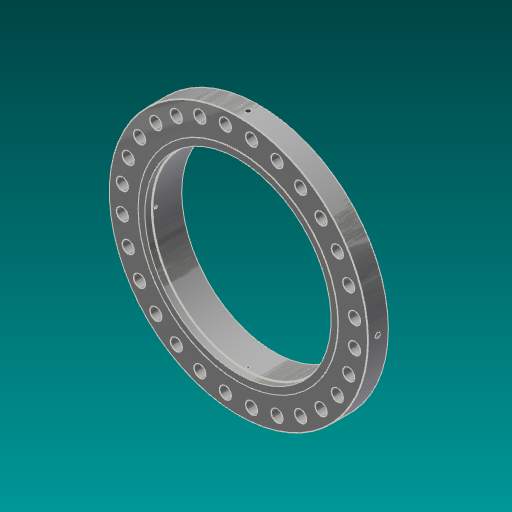
# Autodesk Inventor part: A1-19037-300-04 26in CL300 RF flange - custom
Saved by Autodesk Inventor 2017.3 (Build 213256000, 256)
## iProperties
Created: 2011-05-31
Part Number: A1-19037-300-04 26in CL300 RF flange - custom
Document SubType Name: Modeling
Designer: Graeme_Van_Dongen
Density: 7.85 g/cm^3
Description: 26" CLASS 300 B16.47 Ser.A FFSO FLANGE, A105N, Ø27 1/4" BORE
Material: Steel
Mass: 227317 g
Surface Area: 15864.3 cm^2
Volume: 28957.6 cm^3
Appearance: Steel
Project: A1-19037--CNUL Albian CST laterals
Constructed By: Graeme_Van_Dongen
Project Name: CST laterals
Author: Graeme_Van_Dongen
Autodesk Inventor part; units mm, degrees
ref_plane "YZ Plane" through (0, 0, 0) normal (1, 0, 0) x (0, 1, 0)
ref_plane "XY Plane" through (0, 0, 0) normal (0, 0, 1) x (1, 0, 0)
sketch "Sketch1" plane through (0, 0, 0) normal (0, 0, 1) x (1, 0, 0)
  circle A0 centre (0, 0) radius 485.775
  circle A1 centre (0, 0) radius 346.075
  dimension "d0" = 971.55
  dimension "d1" = 692.15
  constraints: 2 centre point, 2 coincident
  measures "d0" diameter of A0
  measures "d1" diameter of A1
extrude "Extrusion1" add sketch "Sketch1" along normal blind 77.7875
sketch "Sketch2" plane through (0, 0, 77.7875) normal (0, 0, 1) x (1, 0, 0)
  circle A0 centre (0, 0) radius 346.075 projected
  circle A1 centre (0, 0) radius 485.775 projected
  circle A2 centre (0, 0) radius 374.65
  dimension "d4" = 749.3
  constraints: 1 centre point, 1 coincident
  measures "d4" diameter of A2
extrude "Extrusion2" add sketch "Sketch2" along normal blind 1.5875 contours A2
sketch "Sketch3" plane through (0, 0, 0) normal (0, 0, -1) x (-1, 0, 0)
  circle A0 centre (0, 0) radius 346.075 projected
  circle A1 centre (0, 0) radius 485.775 projected
  circle A2 centre (0, 0) radius 384.175
  dimension "d7" = 768.35
  constraints: 1 centre point, 1 coincident
  measures "d7" diameter of A2
extrude "Extrusion3" add sketch "Sketch3" along normal blind 55.5625 contours A2
sketch "Sketch4" plane through (0, 0, 79.375) normal (0, 0, 1) x (1, 0, 0)
  line L0 (0, 0) -> (49.0572, 435.395) construction
  line L1 (0, -681.9981) -> (0, 691.5638) construction
  dimension "d13" = 438.15
  dimension "d99" = 6.429
  constraints: 2 end point
  measures "d13" distance of L0.start L0.end
  measures "d99" angle of L0 L1
hole "Hole1" at (49.0572, 435.395, 79.375) direction (0, 0, -1) diameter 44.45 end through all
chamfer "Chamfer3" distance 0.7937 angle 45 2 edges at (49.0572, 457.62, 0) (49.0572, 457.62, 77.7875)
pattern_circular "Circular Pattern1" count 28 over 360 about axis through (0, 0, -10) along (0, 0, -1) of "Hole1", "Chamfer3"
chamfer "Chamfer2" distance 1.5875 angle 45 2 edges at (-485.775, 0, 0) (-485.775, 0, 77.7875)
fillet "Fillet2" radius 9.525 1 edges at (384.175, 0, 0)
chamfer "Chamfer4" distance 1.5875 angle 45 1 edges at (384.175, 0, -55.5625)
sketch "Sketch6" plane through (0, 0, 0) normal (1, 0, 0) x (0, 1, 0)
  line L0 (384.175, -9.525) -> (384.175, -53.975) construction
  line L1 (382.5875, -55.5625) -> (-382.5875, -55.5625) construction
  line L2 (381, -35.8131) -> (363.5375, -49.2125)
  line L3 (360.3625, -55.5625) -> (384.175, -55.5625)
  line L4 (0, -92.71) -> (0, 122.8725) projected
  line L5 (360.3625, -55.5625) -> (360.3625, -49.2125)
  line L6 (346.075, -55.5625) -> (346.075, 79.375) construction
  line L7 (360.3625, -49.2125) -> (363.5375, -49.2125)
  line L8 (346.075, 79.375) -> (349.25, 79.375)
  line L9 (349.25, 79.375) -> (349.25, 53.975)
  line L10 (349.25, 53.975) -> (346.075, 53.975)
  line L11 (346.075, 53.975) -> (346.075, 79.375)
  line L12 (381, -35.8131) -> (381, -30.1625)
  line L13 (384.175, -21.7622) -> (384.175, -55.5625)
  arc A0 (384.175, -21.7622) -> (381, -30.1625) centre (393.7, -30.1625) ccw
  point P0 (0, 0)
  dimension "d45" = 37.5
  dimension "d59" = 6.35
  dimension "d69" = 17.4625
  dimension "d70" = 3.175
  dimension "d71" = 25.4
  dimension "d72" = 349.25
  dimension "d96" = 381
  dimension "d97" = 12.7
  dimension "d98" = 25.4
  constraints: 21 end point, 3 collinear, 3 parallel, 2 horizontal, 2 point on circle, 2 point on line, 1 centre point, 1 perpendicular, 1 tangent, 1 vertical
  measures "d45" angle of L3 L2
  measures "d59" distance of L3.start L5.end
  measures "d69" horizontal distance of L2.start L2.end
  measures "d70" distance of L5.end L2.end
  measures "d71" distance from line of L6.end L10
  measures "d72" distance from line of point (0, 0) L9
  measures "d96" distance between parallel lines of L4 L12
  measures "d97" radius of A0
  measures "d98" distance from line of A0.centre L3
revolve "Revolution1" cut sketch "Sketch6" angle 360 about axis through (0, 0, -10) along (0, 0, 1)
fillet "Fillet5" radius 0.7937 1 edges at (0, -349.25, 53.975)
chamfer "Chamfer7" distance 0.7937 angle 45 1 edges at (-346.075, 0, 53.975)
ref_plane "Work Plane1" through (0, 485.775, 0) normal (0, 1, 0) x (-1, 0, 0)
sketch "Sketch11" plane through (0, 485.775, 0) normal (0, 1, 0) x (-1, 0, 0)
  line L0 (-348.4563, 53.975) -> (348.4563, 53.975) construction
  line L1 (346.8687, 53.975) -> (-346.8687, 53.975) construction
  point P0 (0, 0)
  point P1 (0, 41.275)
  dimension "d101" = 12.7
  constraints: 1 vertical alignment
  measures "d101" distance from line of L0 point (0, 41.275)
hole "Hole4" at (0, 485.775, 41.275) direction (0, -1, 0) diameter 17.4752 depth 22.6314 tip angle 118 thread size "1/2" designation "1/2 - 14 NPT" standard "NPT"
hole "Hole5" at (0, 485.775, 41.275) direction (0, -1, 0) diameter 10.5918 depth 38.1 tip angle 118 thread size "1/2-13 UNC" class "2B" standard "ANSI Unified Screw Threads"
hole "Hole6" at (0, 485.775, 41.275) direction (0, -1, 0) diameter 10.3188 depth 152.4 tip angle 118
pattern_circular "Circular Pattern3" count 4 over 360 about axis through (0, 0, -10) along (0, 0, 1) of "Hole4", "Hole5", "Hole6"
equation "\"d0\" = OD"
equation "\"d1\" = Bore"
equation "\"d2\" = Thickness"
equation "\"d4\" = RFDia"
equation "\"d5\" = RFDepth"
equation "\"d7\" = NeckDia"
equation "\"d8\" = NeckLength"
equation "\"d13\" = 0.5 * BCD"
equation "\"d15\" = HoleDia"
equation "\"d30\" = HoleChamfer"
equation "\"d25\" = RimChamfer"
equation "\"d29\" = NeckFillet"
equation "\"d33\" = NeckChamfer"
equation "\"d72\" = 0.5 * Bore + Lockstep"
equation "\"d96\" = 0.5 * Casing"
equation "\"OD\" = 971.55"
equation "\"Bore\" = 692.15"
equation "\"Thickness\" = 77.7875"
equation "\"RFDia\" = 749.3"
equation "\"RFDepth\" = 1.5875"
equation "\"HoleDia\" = 44.45"
equation "\"BCD\" = 876.3"
equation "\"NeckDia\" = 768.35"
equation "\"NeckLength\" = 55.5625"
equation "\"HoleChamfer\" = 0.79375"
equation "\"RimChamfer\" = 1.5875"
equation "\"NeckChamfer\" = 1.5875"
equation "\"NeckFillet\" = 9.525"
equation "\"Lock\" = 25.4"
equation "\"Lockstep\" = 3.175"
equation "\"Size\" = 660.4"
equation "\"Wall\" = 19.05"
equation "\"Casing\" = 762"
body "Solid1"
